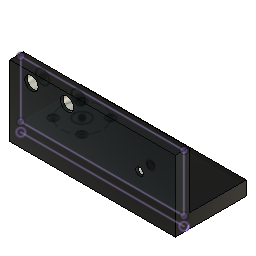
rotoforgeender3mount v4 (Autodesk Fusion 360 design; units mm, degrees)
Autodesk Fusion 360 part; units mm, degrees
note: some values were not read from the file. Chosen so that the rebuilt part matches the saved one: which face or edge a step refers to; where a thread starts.
sketch "Sketch1" plane through (0, 0, 0) normal (1, 0, 0) x (0, 1, 0)
  line L0 (0, 0) -> (0, 22.27)
  line L1 (0, 22.27) -> (-3.35, 22.27)
  line L2 (-3.35, 22.27) -> (-3.35, -3.53)
  line L3 (-3.35, -3.53) -> (22.45, -3.53)
  line L4 (0, 0) -> (22.45, 0)
  line L5 (22.45, 0) -> (22.45, -3.53)
  dimension "d1" = 22.27
  dimension "d2" = 3.35
  dimension "d3" = 25.8
  dimension "d4" = 25.8
  constraint coincident L0.start L4.start
  constraint vertical L0
  constraint perpendicular L0 L1
  constraint perpendicular L1 L2
  constraint perpendicular L2 L3
  constraint perpendicular L0 L4
  constraint perpendicular L3 L5
  measures "d1" distance of L0.start L0.end
  measures "d2" distance of L0.end L1.end
  measures "d3" distance of L1.end L2.end
  measures "d4" distance of L2.end L3.end
extrude "Extrude1" add sketch "Sketch1" along normal blind 64 makes body 1
sketch "Sketch2" plane through (0, 0, 0) normal (0, 1, 0) x (-1, 0, 0)
  line L0 (0, 0) -> (0, 22.27)
  line L1 (0, 22.27) -> (-64, 22.27)
  line L2 (-64, 22.27) -> (-64, 0)
  line L3 (-64, 0) -> (0, 0)
  circle A0 centre (-8.5, 19.52) radius 2.625
  line L4 (0, -3.53) -> (-64, -3.53)
  circle A1 centre (-22.5, 19.52) radius 2.625
  circle A2 centre (-50.93, 10.72) radius 1.5
  dimension "d7" = 5.25
  dimension "d9" = 8.5
  dimension "d10" = 23.05
  dimension "d11" = 5.25
  dimension "d12" = 14
  dimension "d13" = 3
  dimension "d14" = 50.93
  dimension "d15" = 14.25
  constraint horizontal A0.centre A1.centre
  measures "d7" diameter of A0
  measures "d9" distance of L0 A0.centre
  measures "d10" distance of A0.centre L4
  measures "d11" diameter of A1
  measures "d12" distance of A0.centre A1.centre
  measures "d13" diameter of A2
  measures "d14" distance of L0 A2.centre
  measures "d15" distance of L4 A2.centre
extrude "Extrude2" cut sketch "Sketch2" against normal through all contours A0 | A1 | A2 bodies 1
sketch "Sketch3" plane through (0, 0, 0) normal (0, 0, 1) x (-1, 0, 0)
  line L0 (0, -22.45) -> (0, 0)
  line L1 (0, 0) -> (-64, 0)
  line L2 (-64, 0) -> (-64, -22.45)
  line L3 (-64, -22.45) -> (0, -22.45)
  circle A0 centre (-5, -19) radius 1.625
  circle A1 centre (-10.6569, -13.3431) radius 8 construction
  circle A2 centre (-5, -7.6863) radius 1.625
  circle A3 centre (-16.3137, -7.6863) radius 1.625
  circle A4 centre (-16.3137, -19) radius 1.625
  circle A5 centre (-10.6569, -13.3431) radius 3
  dimension "d17" = 3.25
  dimension "d18" = 19
  dimension "d19" = 5
  dimension "d20" = 16
  dimension "d23" = 360
  dimension "d24" = 6
  constraint coincident A0.centre A1
  constraint horizontal A0.centre A4.centre
  constraint concentric A1 A5
  measures "d17" diameter of A0
  measures "d18" distance of L1 A0.centre
  measures "d19" distance of L0 A0.centre
  measures "d20" diameter of A1
  measures "d24" diameter of A5
hole "Hole1" at (10.6569, 13.3431, 0) direction (0, 0, -1) diameter 5.035 end through all bodies 1
thread "Thread1" "ISO Metric profile 6.0 M6x1 6H" major diameter 6.147 minor diameter 5.035 pitch 1 angle 60 modelled right hand crest width 0.2748 on face at (10.9075, 10.8382, -1.1767) crest through (10.6569, 10.8256, 0.5) on bodies 1
extrude "Extrude3" cut sketch "Sketch3" against normal through all contours A0 | A2 | A3 | A4 bodies 1
sketch "Sketch4" plane through (0, 0, 0) normal (-1, 0, 0) x (0, -1, 0)
  line L0 (0, 22.27) -> (0, 0)
  line L1 (0, 0) -> (-22.45, 0)
  line L2 (-22.45, 0) -> (-22.45, -3.53)
  line L3 (-22.45, -3.53) -> (3.35, -3.53)
  line L4 (3.35, -3.53) -> (3.35, 22.27)
  line L5 (3.35, 22.27) -> (0, 22.27)
  line L6 (1, 23.27) -> (4.35, 23.27)
  line L7 (4.35, 23.27) -> (4.35, -4.53)
  line L8 (4.35, -4.53) -> (-23.45, -4.53)
  line L9 (-23.45, -4.53) -> (-23.45, 1)
  line L10 (-23.45, 1) -> (-1, 1)
  line L11 (-1, 1) -> (-1, 23.27)
  line L12 (-1, 23.27) -> (1, 23.27)
  dimension "d31" = 1
  dimension "d32" = 1
  dimension "d33" = 1
  dimension "d34" = 1
  dimension "d35" = 1
  dimension "d36" = 1
  constraint horizontal L6
  constraint perpendicular L6 L7
  constraint perpendicular L7 L8
  constraint perpendicular L8 L9
  constraint perpendicular L9 L10
  constraint perpendicular L10 L11
  constraint perpendicular L11 L12
  measures "d31" distance of L1 L10
  measures "d32" distance of L0 L11
  measures "d33" distance of L4 L7
  measures "d34" distance of L3 L8
  measures "d35" distance of L2 L9
  measures "d36" distance of L5 L12
extrude "Extrude4" add sketch "Sketch4" against normal blind 64 separate body makes body 2
sketch "Sketch5" plane through (0, 0, 1) normal (0, 0, 1) x (-1, 0, 0)
  line L0 (0, -23.45) -> (0, -1)
  line L1 (0, -1) -> (-64, -1)
  line L2 (-64, -1) -> (-64, -23.45)
  line L3 (-64, -23.45) -> (0, -23.45)
  circle A0 centre (-16.3137, -7.6863) radius 1.625
  circle A1 centre (-10.6569, -13.3431) radius 3
  circle A2 centre (-5, -7.6863) radius 1.625
  circle A3 centre (-5, -19) radius 1.625
  circle A4 centre (-16.3137, -19) radius 1.625
extrude "Extrude5" cut sketch "Sketch5" against normal through all contours A0 | A1 | A2 | A3 | A4 bodies 2
sketch "Sketch6" plane through (0, 1, 0) normal (0, 1, 0) x (-1, 0, 0)
  line L0 (0, 1) -> (0, 23.27)
  line L1 (0, 23.27) -> (-64, 23.27)
  line L2 (-64, 23.27) -> (-64, 1)
  line L3 (-64, 1) -> (0, 1)
  line L4 (0, 22.27) -> (0, 0)
  line L5 (0, 0) -> (0, -3.53)
  line L6 (0, -3.53) -> (0, 22.27)
  circle A0 centre (-22.5, 19.52) radius 2.625
  circle A1 centre (-8.5, 19.52) radius 2.625
  circle A2 centre (-50.93, 10.72) radius 1.5
extrude "Extrude6" cut sketch "Sketch6" against normal through all contours A0 | A1 | A2 bodies 2
sketch "Sketch7" plane through (64, 0, 0) normal (1, 0, 0) x (0, 1, 0)
  line L0 (-3.35, 22.27) -> (0, 22.27)
  line L1 (0, 22.27) -> (0, 0)
  line L2 (0, 0) -> (22.45, 0)
  line L3 (22.45, 0) -> (22.45, -3.53)
  line L4 (22.45, -3.53) -> (-3.35, -3.53)
  line L5 (-3.35, -3.53) -> (-3.35, 22.27)
  line L6 (1, 1) -> (1, 23.27)
  line L7 (1, 23.27) -> (-4.35, 23.27)
  line L8 (-4.35, 23.27) -> (-4.35, -4.53)
  line L9 (-4.35, -4.53) -> (23.45, -4.53)
  line L10 (23.45, -4.53) -> (23.45, 1)
  line L11 (23.45, 1) -> (1, 1)
  line L12 (0, 0) -> (0, 22.27)
  line L13 (0, 22.27) -> (-3.35, 22.27)
  line L14 (-3.35, 22.27) -> (-3.35, -3.53)
  line L15 (-3.35, -3.53) -> (22.45, -3.53)
  line L16 (22.45, -3.53) -> (22.45, 0)
  line L17 (22.45, 0) -> (0, 0)
extrude "Extrude7" add sketch "Sketch7" along normal blind 1 contours L0 L1 L2 L3 L4 L5 L12 L13 L14 L15 L16 L17 | L6 L7 L8 L9 L10 L11 bodies 2
equation "d9 = 5.875 mm + ( 5.25 / 2 ) * 1 mm"
named bodies: "aluminumanglemount", "drilltemplate"
